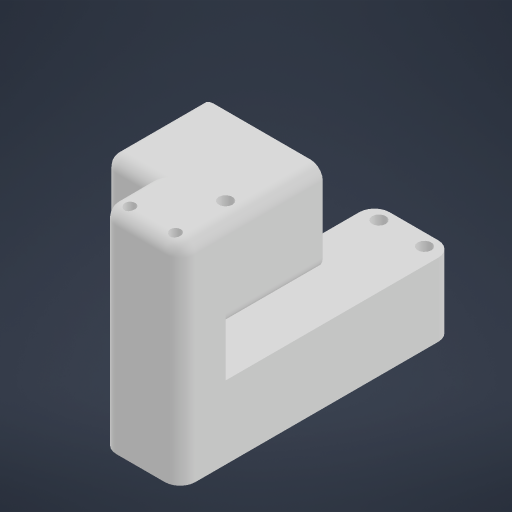
# Autodesk Inventor part: button_holder
Saved by Autodesk Inventor 2024.1 (Build 281209000, 209)
## iProperties
Created: 2025-01-18
Part Number: button_holder
Material: Generic
Document SubType Name: Modeling
Designer: Vibhu Iyer
Density: 1 g/cm^3
Appearance: Default
Author: Vibhu Iyer
Autodesk Inventor part; units mm, degrees
ref_plane "YZ Plane" through (0, 0, 0) normal (1, 0, 0) x (0, 1, 0)
ref_plane "XZ Plane" through (0, 0, 0) normal (0, 1, 0) x (-1, 0, 0)
ref_plane "XY Plane" through (0, 0, 0) normal (0, 0, 1) x (1, 0, 0)
sketch "Sketch1" plane through (0, 0, 0) normal (0, 1, 0) x (-1, 0, 0)
  line L0 (0, 0) -> (22, 0)
  line L1 (22, 0) -> (22, -70)
  line L2 (22, -70) -> (0, -70)
  line L3 (0, -70) -> (0, 0)
  line L4 (24, -72) -> (24, 2)
  line L5 (24, 2) -> (-2, 2)
  line L6 (-2, 2) -> (-2, -72)
  line L7 (-2, -72) -> (24, -72)
  circle A0 centre (18.5, -76) radius 2.25
  circle A1 centre (3.5, -76) radius 2.25
  line L8 (24, -72) -> (-2, -72)
  line L9 (-2, -72) -> (-2, -80)
  line L10 (-2, -80) -> (24, -80)
  line L11 (24, -80) -> (24, -72)
  line L12 (18.5, -76) -> (3.5, -76) construction
  line L13 (22, -35) -> (0, -35) construction
  circle A2 centre (18.5, 6) radius 2.25
  circle A3 centre (3.5, 6) radius 2.25
  line L14 (-2, 2) -> (-2, 10)
  line L15 (-2, 10) -> (24, 10)
  line L16 (24, 10) -> (24, 2)
  line L17 (15, 0) -> (7, 0)
  line L18 (7, 0) -> (7, 8)
  line L19 (7, 8) -> (15, 8)
  line L20 (15, 8) -> (15, 0)
  circle A4 centre (18.5, 6) radius 1.75
  circle A5 centre (3.5, 6) radius 1.75
  point P0 (24, -76)
  point P1 (11, -76)
  point P2 (11, -80)
  point P3 (11, 8)
  point P4 (11, 10)
  point P5 (7, 0)
  dimension "d0" = 22
  dimension "d1" = 70
  dimension "d2" = 2
  dimension "d3" = 4.5
  dimension "d4" = 8
  dimension "d6" = 15
  dimension "d11" = 8
  dimension "d12" = 8
  dimension "d16" = 3.5
  constraints: 42 end point, 8 parallel, 7 midpoint, 6 centre point, 5 symmetric about line, 4 horizontal, 4 perpendicular, 2 coincident, 2 equal radius, 2 horizontal alignment, 2 vertical alignment, 1 collinear, 1 point on line, 5 other
  measures "d0" distance of L1.end L2.end
  measures "d1" distance of L0.end L1.end
  measures "d2" distance between parallel lines of L1 L4
  measures "d3" diameter of A0
  measures "d4" distance between parallel lines of L10 L7
  measures "d6" distance of L12.start L12.end
  measures "d11" distance between parallel lines of L18 L20
  measures "d12" distance between parallel lines of L0 L19
  measures "d16" diameter of A5
extrude "Extrusion1" add sketch "Sketch1" along normal blind 2 contours L3 L2 L1 L0 L20 L5 L4 L7 L6 L18 | L0 L1 L2 L3 | L5 L14 L15 L16 L20 L19 L18 | L7 L11 L10 L9 | A2 | A3
extrude "Extrusion2" add sketch "Sketch1" against normal blind 22 contours L3 L2 L1 L0 L20 L5 L4 L7 L6 L18 | L18 L5 L20 L0 | L18 L19 L20 L5 | L5 L14 L15 L16 L20 L19 L18 | L7 L11 L10 L9
extrude "Extrusion3" cut sketch "Sketch1" against normal blind 34.25 contours L18 L5 L20 L0 | L18 L19 L20 L5
fillet "Fillet1" radius 5 4 edges at (-24, -10, -80) (2, -10, -80) (-24, -10, 10) (2, -10, 10)
sketch "Sketch2" plane through (0, 2, 0) normal (0, 1, 0) x (1, 0, 0)
  arc A0 (-3, -10) -> (2, -5) centre (-3, -5) ccw projected
  line L0 (2, -5) -> (2, 75) projected
  arc A1 (2, 75) -> (-3, 80) centre (-3, 75) ccw projected
  line L1 (-3, 80) -> (-19, 80) projected
  arc A2 (-19, 80) -> (-24, 75) centre (-19, 75) ccw projected
  line L2 (-24, 75) -> (-24, -5) projected
  arc A3 (-24, -5) -> (-19, -10) centre (-19, -5) ccw projected
  line L3 (-19, -10) -> (-3, -10) projected
  line L4 (-15, -8) -> (-15, 0) projected
  line L5 (-15, 0) -> (-7, 0) projected
  line L6 (-7, 0) -> (-7, -8) projected
  line L7 (-7, -8) -> (-15, -8) projected
  circle A4 centre (-3.5, 76) radius 2.25 projected
  circle A5 centre (-18.5, 76) radius 2.25 projected
  line L8 (-24, 5) -> (2, 5)
  circle A6 centre (-18.5, -6) radius 1.75 projected
  circle A7 centre (-3.5, -6) radius 1.75 projected
  point P0 (0, 0)
  dimension "d17" = 15
  constraints: 2 end point, 2 point on line, 1 perpendicular
  measures "d17" distance between parallel lines of L8 L3
extrude "Extrusion4" add sketch "Sketch2" along normal blind 45 contours L3 A3 L2 L8 L0 A0
sketch "Sketch3" plane through (2, 2, -5) normal (0, 0, -1) x (-1, 0, 0)
  line L0 (0, -24) -> (0, 45) projected
  line L1 (0, 45) -> (40, 45)
  line L2 (40, 45) -> (40, 15)
  line L3 (40, 15) -> (0, 15)
  line L4 (0, 15) -> (0, 45)
  line L5 (38, 43) -> (2, 43)
  line L6 (2, 43) -> (2, 17)
  line L7 (2, 17) -> (38, 17)
  line L8 (38, 17) -> (38, 43)
  circle A0 centre (6.25, 38.75) radius 2.25
  circle A1 centre (33.75, 38.75) radius 2.25
  circle A2 centre (33.75, 21.25) radius 2.25
  circle A3 centre (6.25, 21.25) radius 2.25
  circle A4 centre (6.25, 38.75) radius 4.25
  circle A5 centre (33.75, 38.75) radius 4.25
  circle A6 centre (33.75, 21.25) radius 4.25
  circle A7 centre (6.25, 21.25) radius 4.25
  line L9 (6.25, 38.75) -> (33.75, 38.75) construction
  line L10 (33.75, 38.75) -> (33.75, 21.25) construction
  line L11 (33.75, 21.25) -> (6.25, 21.25) construction
  line L12 (6.25, 21.25) -> (6.25, 38.75) construction
  line L13 (10.5, 17) -> (10.5, 43)
  line L14 (29.5, 17) -> (29.5, 43)
  line L15 (38, 25.5) -> (2, 25.5)
  line L16 (2, 34.5) -> (38, 34.5)
  point P0 (2, -2)
  point P1 (20, 30)
  point P2 (20, 15)
  point P3 (0, 30)
  point P4 (0, 15)
  point P5 (38, 21.25)
  point P6 (33.75, 17)
  point P7 (6.25, 17)
  point P8 (2, 21.25)
  point P9 (33.75, 43)
  point P10 (38, 38.75)
  point P11 (2, 38.75)
  point P12 (6.25, 43)
  point P13 (33.75, 25.5)
  point P14 (29.5, 21.25)
  point P15 (29.5, 38.75)
  point P16 (33.75, 34.5)
  point P17 (6.25, 34.5)
  point P18 (10.5, 38.75)
  point P19 (10.5, 21.25)
  point P20 (6.25, 25.5)
  dimension "d23" = 40
  dimension "d26" = 30
  dimension "d27" = 2
  dimension "d32" = 4.5
  dimension "d33" = 2
  constraints: 32 end point, 8 centre point, 8 point on line, 8 tangent, 7 perpendicular, 6 coincident, 6 equal radius, 6 parallel, 2 horizontal, 2 midpoint, 3 other
  measures "d23" distance of L2.end L3.end
  measures "d26" distance between parallel lines of L3 L1
  measures "d27" distance between parallel lines of L1 L5
  measures "d32" diameter of A1
  measures "d33" radial gap between concentric circles of A2 A6
extrude "Extrusion5" add sketch "Sketch3" along normal blind 2 contours L0 L1 L2 L3 | L14 L16 L13 L5 | L5 A5 L14 | L13 A4 L5 | L5 L8 A5 | A5 | A5 L16 L14 | A4 L6 L5 | A4 | L13 L16 A4 | L8 L16 A5 | L16 L8 L15 L14 | L14 L15 L13 L16 | A4 L16 L6 | L16 L13 L15 L6 | L15 A6 L14 | L14 L7 L13 L15 | L13 A7 L15 | L8 A6 L15 | A6 | A6 L7 L14 | L15 A7 L6 | A7 | L13 L7 A7 | L8 L7 A6 | A7 L7 L6 | A0 | A1 | A2 | A3
extrude "Extrusion6" add sketch "Sketch3" along normal blind 30 from surface at 2 contours L0 L1 L2 L3
sketch "Sketch5" plane through (0, 47, 0) normal (0, 1, 0) x (1, 0, 0)
  line L0 (-36, 7) -> (0, 7) projected
  line L1 (-36, 37) -> (-36, 7) projected
  line L2 (-36, 37) -> (0, 37) projected
  line L3 (0, 7) -> (0, 37) projected
  circle A0 centre (-4.25, 11.25) radius 2.25
  circle A1 centre (-4.25, 11.25) radius 4.25
  line L4 (0, 7) -> (-8.5, 7)
  line L5 (-8.5, 7) -> (-8.5, 15.5)
  line L6 (-8.5, 15.5) -> (0, 15.5)
  line L7 (0, 15.5) -> (0, 7)
  point P0 (0, 0)
  point P1 (0, 11.25)
  point P2 (-4.25, 7)
  point P3 (0, 15.5)
  point P4 (-4.25, 15.5)
  point P5 (-8.5, 11.25)
  dimension "d36" = 2
  dimension "d37" = 4.5
  constraints: 8 end point, 4 tangent, 2 centre point, 2 parallel, 1 coincident, 1 horizontal, 1 perpendicular
  measures "d36" radial gap between concentric circles of A1 A0
  measures "d37" diameter of A0
extrude "Extrusion8" add sketch "Sketch5" against normal up to surface (28 mm away) contours L5 A1 L0 | A1 L3 L0 | A1 | A1 L6 L3
extrude "Extrusion13" add sketch "Sketch3" against normal up to surface (21.5 mm away) from surface at 32 contours L13 A4 L5 | A4 L6 L5 | A4 | A4 L16 L6 | L15 A7 L6 | A7 | L13 L7 A7 | A7 L7 L6
extrude "Extrusion14" add sketch "Sketch3" against normal up to surface from surface at 10.5 contours L13 A4 L5 | A4 L6 L5 | A4 | A4 L16 L6 | L15 A7 L6 | A7 | L13 L7 A7 | A7 L7 L6 round surface about axis through (-4.25, 47, -11.25) along (0, -1, 0) radius 4.25 far side no
extrude "Extrusion15" add sketch "Sketch3" against normal up to surface (30 mm away) from surface at 32 contours L5 A5 L14 | L5 L8 A5 | A5 | L8 L16 A5 | L8 A6 L15 | A6 | A6 L7 L14 | L8 L7 A6
extrude "Extrusion9" cut sketch "Sketch5" against normal up to surface (45 mm away) contours A0
sketch "Sketch6" plane through (2, 2, -7) normal (0, 0, -1) x (-1, 0, 0)
  line L0 (9, -24) -> (9, 45) projected
  line L1 (17, -24) -> (9, -24) projected
  line L2 (17, 45) -> (17, -24) projected
  line L3 (9, 45) -> (17, 45) projected
  line L4 (17, -2) -> (17, 45) projected
  line L5 (9, -2) -> (9, 45) projected
  line L6 (17, 35) -> (9, 35)
  line L7 (9, 35) -> (9, 25)
  line L8 (9, 25) -> (17, 25)
  line L9 (17, 25) -> (17, 35)
  line L10 (38, 17) -> (38, 43) projected
  point P0 (2, -2)
  point P1 (38, 21.25)
  point P2 (38, 38.75)
  point P3 (17, 30)
  point P4 (38, 30)
  point P5 (9, 25)
  point P6 (17, 25)
  point P7 (17, 35)
  point P8 (9, 35)
  point P9 (38, 25.5)
  point P10 (38, 34.5)
  dimension "d42" = 10
  constraints: 8 end point, 2 midpoint, 2 parallel, 2 point on line, 1 horizontal, 1 horizontal alignment, 1 perpendicular
  measures "d42" distance between parallel lines of L8 L6
extrude "Extrusion10" cut sketch "Sketch6" against normal up to surface (7 mm away) contours L0 L6 L2 L8
sketch "Sketch7" plane through (0, 47, 0) normal (0, 1, 0) x (1, 0, 0)
  line L0 (-7, 0) -> (-7, -8) projected
  line L1 (-15, -8) -> (-15, 0) projected
  line L2 (-15, 0) -> (-7, 0) projected
  line L3 (-7, -8) -> (-15, -8) projected
  point P0 (0, 0)
extrude "Extrusion12" add sketch "Sketch7" against normal up to surface (10 mm away)
fillet "Fillet2" radius 4 10 edges at (0.5355, 47, 8.5355) (-11, 47, 10) (-22.5355, 47, 8.5355) (-24, 47, 0) (2, 47, -16) (-38, 47, -21) (-31, 47, -5) (2, 17, -21) (-38, 17, -21) (-38, 32, -5)
fillet "Fillet3" radius 4 2 edges at (-7, 7.5, 8) (-15, 7.5, 8)
body "Solid1"
